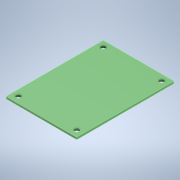
# Autodesk Inventor part: rpcomputemodule4
Saved by Autodesk Inventor 2022 (Build 260153000, 153)
## iProperties
Created: 2021-10-07
Part Number: rpcomputemodule4
Material: Generic
Document SubType Name: Modeling
Designer: Bowen O'Steen
Density: 1 g/cm^3
Appearance: Smooth - Dark Forest Green
Author: Bowen O'Steen
Autodesk Inventor part; units mm, degrees
ref_plane "YZ Plane" through (0, 0, 0) normal (1, 0, 0) x (0, 1, 0)
ref_plane "XZ Plane" through (0, 0, 0) normal (0, 1, 0) x (-1, 0, 0)
ref_plane "XY Plane" through (0, 0, 0) normal (0, 0, 1) x (1, 0, 0)
sketch "Sketch1" plane through (0, 0, 0) normal (0, 1, 0) x (-1, 0, 0)
  line L0 (20, 27.5) -> (-20, 27.5)
  line L1 (-20, 27.5) -> (-20, -27.5)
  line L2 (-20, -27.5) -> (20, -27.5)
  line L3 (20, -27.5) -> (20, 27.5)
  point P0 (0, 0)
  point P1 (20, 0)
  point P2 (0, -27.5)
  dimension "d0" = 55
  dimension "d1" = 40
  constraints: 8 end point, 2 midpoint, 2 parallel, 1 horizontal, 1 horizontal alignment, 1 perpendicular, 1 vertical alignment
  measures "d0" distance of L2.end L0.start
  measures "d1" distance of L1.end L2.end
extrude "Extrusion1" add sketch "Sketch1" along normal blind 1.2
sketch "Sketch2" plane through (0, 1.2, 0) normal (0, 1, 0) x (1, 0, 0)
  line L0 (-20, 27.5) -> (-20, -27.5) projected
  line L1 (20, -27.5) -> (20, 27.5) projected
  line L2 (-20, -27.5) -> (20, -27.5) projected
  line L3 (20, 27.5) -> (-20, 27.5) projected
  point P0 (0, 0)
  point P1 (-16.5, -24)
  point P2 (-16.5, 24)
  point P3 (16.5, -24)
  point P4 (16.5, 24)
  dimension "d4" = 3.5
  dimension "d5" = 3.5
  dimension "d6" = 3.5
  dimension "d7" = 3.5
  constraints: 2 horizontal alignment, 2 vertical alignment
  measures "d4" distance from line of L0 point (-16.5, -24)
  measures "d5" distance from line of L1 point (16.5, -24)
  measures "d6" distance from line of L2 point (16.5, -24)
  measures "d7" distance from line of L3 point (16.5, 24)
hole "Hole1" at (-16.5, 1.2, 24) at (-16.5, 1.2, -24) at (16.5, 1.2, 24) at (16.5, 1.2, -24) direction (0, -1, 0) diameter 2.7 end through all clearance for "Flat Head Machine Screw" size "M2.5" standard "Ansi Metric M Profile"
body "Solid1"
